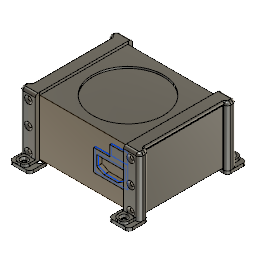
PSU (Autodesk Fusion 360 design; units mm, degrees)
Autodesk Fusion 360 part; units mm, degrees
sketch "Sketch1" plane through (0, 0, 0) normal (0, 0, 1) x (1, 0, 0)
  line L0 (50, 50) -> (-50, 50) construction
  line L1 (-50, 50) -> (-50, -50) construction
  line L2 (-50, -50) -> (50, -50) construction
  line L3 (50, -50) -> (50, 50) construction
  line L4 (50, 50) -> (-50, -50) construction
  line L5 (-50, 50) -> (50, -50) construction
  circle A0 centre (-50, -50) radius 2.25
  circle A1 centre (-50, -50) radius 3.75
  circle A2 centre (50, -50) radius 3.75
  circle A3 centre (50, -50) radius 2.25
  circle A4 centre (50, 50) radius 3.75
  circle A5 centre (50, 50) radius 2.25
  circle A6 centre (-50, 50) radius 3.75
  circle A7 centre (-50, 50) radius 2.25
  line L6 (63, 50.5) -> (-63, 50.5) construction
  line L7 (-63, 50.5) -> (-63, -50.5)
  line L8 (-63, -50.5) -> (63, -50.5)
  line L9 (63, -50.5) -> (63, 50.5) construction
  line L10 (63, 50.5) -> (-63, -50.5) construction
  line L11 (-63, 50.5) -> (63, -50.5) construction
  line L12 (-50, -50) -> (-63, -50) construction
  line L13 (-56.5, -50) -> (-56.5, -61) construction
  circle A8 centre (-56.5, -61) radius 2.25
  line L14 (-56.5, -61) -> (-50, -50) construction
  line L15 (-48.4461, -44.5539) -> (-64, -44.5539)
  line L16 (-68, -48.5539) -> (-68, -62.9425)
  line L17 (-64, -66.9425) -> (-48.4461, -66.9425)
  line L18 (-44.4461, -62.9425) -> (-44.4461, -48.5539)
  arc A9 (-68, -62.9425) -> (-64, -66.9425) centre (-64, -62.9425) ccw
  arc A10 (-44.4461, -48.5539) -> (-48.4461, -44.5539) centre (-48.4461, -48.5539) ccw
  arc A11 (-48.4461, -66.9425) -> (-44.4461, -62.9425) centre (-48.4461, -62.9425) ccw
  arc A12 (-64, -44.5539) -> (-68, -48.5539) centre (-64, -48.5539) ccw
  line L19 (-56.4568, -56.7278) -> (-60.1782, -58.8265)
  line L20 (-60.1782, -58.8265) -> (-60.2214, -63.0987)
  line L21 (-60.2214, -63.0987) -> (-56.5432, -65.2722)
  line L22 (-56.5432, -65.2722) -> (-52.8218, -63.1735)
  line L23 (-52.8218, -63.1735) -> (-52.7786, -58.9013)
  line L24 (-52.7786, -58.9013) -> (-56.4568, -56.7278)
  circle A13 centre (-50, -50) radius 4.5
  point P0 (-53.25, -55.5)
  point P1 (-53.25, -55.5)
  point P2 (-56.5, -61)
  dimension "d1" = 100
  dimension "d2" = 100
  dimension "d3" = 4.5
  dimension "d4" = 7.5
  dimension "d6" = 360
  dimension "d7" = 126
  dimension "d8" = 101
  dimension "d9" = 11
  dimension "d10" = 4.5
  dimension "d11" = 4
  dimension "d12" = 3.7
  dimension "d23" = 5
  dimension "d24" = 9
  constraint perpendicular L0 L1
  constraint parallel L0 L2
  constraint parallel L1 L3
  constraint horizontal L0
  constraint coincident L4 origin
  constraint coincident L5 origin
  constraint coincident L1.end L2.start
  constraint concentric A0 A1
  constraint perpendicular L6 L7
  constraint parallel L6 L8
  constraint parallel L7 L9
  constraint horizontal L6
  constraint coincident L10 origin
  constraint coincident L11 origin
  constraint coincident L7 L12.end
  constraint perpendicular L7 L12
  constraint midpoint L12 L13.start
  constraint perpendicular L8 L13
  constraint coincident P2 L13.end
  constraint midpoint L14 P1
  constraint perpendicular L15 L16
  constraint parallel L15 L17
  constraint parallel L16 L18
  constraint horizontal L15
  constraint coincident P1 P0
  constraint tangent L16 A9
  constraint tangent L17 A9
  constraint tangent L15 A10
  constraint tangent L18 A10
  constraint equal A9 A10
  constraint tangent L18 A11
  constraint tangent L17 A11
  constraint equal A9 A11
  constraint tangent L15 A12
  constraint tangent L16 A12
  constraint equal A9 A12
  measures "d1" distance of L1.end L2.end
  measures "d2" distance of L0.end L1.end
  measures "d3" diameter of A0
  measures "d4" diameter of A1
  measures "d7" distance of L7.end L8.end
  measures "d8" distance of L6.end L7.end
  measures "d9" distance of L13.start P2
  measures "d10" diameter of A8
  measures "d11" radius of A9
  measures "d12" distance of P2 L24
  measures "d23" distance of L7 L16
  measures "d24" diameter of A13
extrude "Extrude1" add sketch "Sketch1" against normal blind 1 contours A1 L8 A13 | A1 L8 A13 | L7 L8 L15 L16 L17 L18 A9 A11 A12 A13 | L7 L8 L15 L18 A10 A13 makes body 1
extrude "Extrude2" add sketch "Sketch1" along normal blind 1 contours A0 A1 L8 | A0 A1 L8 | A1 L8 A13 | A1 L8 A13 | L7 L8 L15 L16 L17 L18 A9 A11 A12 A13 | L7 L8 L15 L18 A10 A13 bodies 1
extrude "Extrude3" add sketch "Sketch1" along normal blind 1.5 from surface at 1 contours L7 L8 L15 L16 L17 L18 A9 A11 A12 A13 | L7 L8 L15 L18 A10 A13 | L19 L20 L21 L22 L23 L24 bodies 1
mirror "Mirror1" about plane through (0, 0, 0) normal (0, 1, 0) of bodies 1 makes body 2
sketch "Sketch2" plane through (0, 0, 2.5) normal (0, 0, 1) x (-1, 0, 0)
  circle A0 centre (56.5, 61) radius 2.25
  circle A1 centre (50, 50) radius 4.5
  arc A2 (64, 44.5539) -> (68, 48.5539) centre (64, 48.5539) ccw
  line L0 (68, 48.5539) -> (68, 62.9425)
  arc A3 (68, 62.9425) -> (64, 66.9425) centre (64, 62.9425) ccw
  line L1 (64, 66.9425) -> (48.4461, 66.9425)
  arc A4 (48.4461, 66.9425) -> (44.4461, 62.9425) centre (48.4461, 62.9425) ccw
  line L2 (44.4461, 62.9425) -> (44.4461, 48.5539)
  arc A5 (44.4461, 48.5539) -> (48.4461, 44.5539) centre (48.4461, 48.5539) ccw
  line L3 (48.4461, 44.5539) -> (64, 44.5539)
  line L4 (63, -50.5) -> (63, 50.5)
  line L5 (63, 50.5) -> (-63, 50.5)
  line L6 (54.9957, 66.9425) -> (57.9957, 66.9425)
  line L7 (62.9957, 61.9425) -> (62.9957, 56.0653)
  line L8 (49.9957, 55.0496) -> (49.9957, 61.9425)
  line L9 (49.9957, 66.9425) -> (62.9957, 55.0653) construction
  line L10 (62.9957, 66.9425) -> (49.9957, 55.0496) construction
  line L11 (64, 66.9425) -> (48.4461, 66.9425)
  line L12 (63.9957, 55.0653) -> (63.9997, 55.0653)
  line L13 (49.9957, 55.0496) -> (49.9957, 50.5)
  arc A6 (62.9957, 56.0653) -> (63.9957, 55.0653) centre (63.9957, 56.0653) ccw
  line L14 (67.9997, 51.0657) -> (68, 48.5539)
  arc A7 (67.9997, 51.0657) -> (63.9997, 55.0653) centre (63.9997, 51.0653) ccw
  arc A8 (62.9957, 61.9425) -> (57.9957, 66.9425) centre (57.9957, 61.9425) ccw
  arc A9 (54.9957, 66.9425) -> (49.9957, 61.9425) centre (54.9957, 61.9425) ccw
  line L15 (63.9997, 55.0653) -> (49.9957, 55.0496)
  point P0 (56.5, 61)
  dimension "d25" = 13
  dimension "d26" = 1
  dimension "d27" = 4
  dimension "d28" = 5
  constraint perpendicular L6 L7
  constraint parallel L7 L8
  constraint horizontal L6
  constraint coincident L9 P0
  constraint coincident L10 P0
  constraint coincident P0 A0.centre
  constraint collinear L6 L11
  constraint perpendicular L0 L12
  constraint coincident L5 L13.end
  constraint perpendicular L5 L13
  constraint coincident L9.end L12
  constraint coincident L9.end L7
  constraint tangent L12 A6
  constraint tangent L7 A6
  constraint coincident A2.end L0.start
  constraint tangent L12 A7
  constraint tangent L14 A7
  constraint coincident L10.start L7
  constraint coincident L10.start L6
  constraint tangent L7 A8
  constraint tangent L6 A8
  constraint coincident L9.start L8
  constraint coincident L9.start L6
  constraint tangent L8 A9
  constraint tangent L6 A9
  constraint equal A8 A9
  measures "d25" distance of L9.end L8.start
  measures "d26" radius of A6
  measures "d27" radius of A7
  measures "d28" radius of A8
extrude "Extrude4" add sketch "Sketch2" along normal blind 3 separate body contours A1 L5 L13 | A1 A2 L0 L3 L4 L5 L12 L13 L14 A7 L15 | L1 L6 L7 L8 L11 A6 A8 A9 L15 picked at (52.9399, 50.7152) makes body 3
extrude "Extrude5" add sketch "Sketch2" along normal blind 67 contours A1 L5 L13 | A1 A2 L0 L3 L4 L5 L12 L13 L14 A7 L15 picked at (52.9399, 50.7152) bodies 3
mirror "Mirror2" about plane through (0, 0, 0) normal (0, 1, 0) of bodies 3 makes body 4
sketch "Sketch3" plane through (0.0616, -54.9935, 0) normal (0.001121, -0.999999, 0) x (0.999999, 0.001121, 0)
  line L0 (-64.0574, 5.5) -> (-50.0574, 5.5)
  line L1 (-50.0574, 5.5) -> (-50.0574, 69.5)
  line L2 (-50.0574, 69.5) -> (-64.0614, 69.5)
  line L3 (-64.0614, 69.5) -> (-64.0614, 2.5)
  line L4 (-50.0574, 69.5) -> (-64.0614, 69.5)
  line L5 (-64.0614, 69.5) -> (-64.0614, 66.5)
  line L6 (-64.0614, 66.5) -> (-50.0574, 66.5)
  line L7 (-50.0574, 66.5) -> (-50.0574, 69.5)
  line L8 (-58.0614, 66.5) -> (-58.0614, 5.5) construction
  circle A0 centre (-58.0614, 60.5) radius 2.25
  circle A1 centre (-58.0614, 34.7) radius 2.25
  circle A2 centre (-58.0614, 9) radius 2.25
  line L9 (-64.0574, 2.5) -> (-64.0574, 5.5)
  line L10 (-64.0614, 2.5) -> (-64.0574, 2.5)
  dimension "d34" = 3
  dimension "d37" = 6
  dimension "d38" = 4.5
  dimension "d39" = 4.5
  dimension "d40" = 4.5
  dimension "d41" = 6
  dimension "d42" = 25.8
  dimension "d43" = 51.5
  constraint horizontal L4
  constraint vertical L5
  constraint horizontal L6
  constraint vertical L7
  constraint coincident L1.end L2.start
  constraint coincident L6 L8.start
  constraint coincident L0 L8.end
  constraint perpendicular L0 L8
  constraint coincident L8 A0.centre
  constraint coincident L8 A1.centre
  constraint coincident L8 A2.centre
  measures "d34" distance of L1.end L6.end
  measures "d37" distance of L3 L8
  measures "d38" diameter of A0
  measures "d39" diameter of A1
  measures "d40" diameter of A2
  measures "d41" distance of L6 A0.centre
  measures "d42" distance of A0.centre A1.centre
  measures "d43" distance of A0.centre A2.centre
extrude "Extrude6" add sketch "Sketch3" against normal blind 110 contours L1 L2 L3 L4 L5 L6 L7 bodies 3 4
extrude "Extrude7" cut sketch "Sketch3" against normal blind 10 contours A0 | A1 | A2 bodies 3
fillet "Fillet1" radius 3 4 edges at (-66.8325, -45.7295, 69.5) (-67.9999, -49.8098, 69.5) (-66.828, -53.8939, 69.5) (-56.9977, -55.0575, 69.5) on bodies 3
fillet "Fillet1" radius 2 1 edges at (-64.0614, 0.0008, 69.5) on bodies 3
fillet "Fillet1" radius 3 4 edges at (-66.8675, 45.7651, 69.5) (-67.9999, 49.8098, 69.5) (-66.828, 53.8939, 69.5) (-56.9977, 55.0575, 69.5) on bodies 3
chamfer "Chamfer1" distance 2 angle 45 5 edges at (-54.4023, -61.8136, 5.5) (-60.0975, -55.0609, 9.8136) (-60.0975, -55.0609, 35.5136) (-60.0975, -55.0609, 61.3136) (-54.4023, 61.8136, 5.5) on bodies 3 4
mirror "Mirror3" about plane through (0, 0, 0) normal (1, 0, 0) of bodies 3 1 2 makes body 5 at (54.0272, 15.0364, 66.5) makes body 6 at (64.7863, 57.0763, 2.5) makes body 7 at (64.7863, -57.0763, 2.5)
sketch "Sketch4" plane through (0, 0, 66.5) normal (0, 0, -1) x (1, 0, 0)
  arc A0 (-64, -44.5539) -> (-64.1114, -44.5555) centre (-64, -48.5539) ccw
  line L0 (-64, -44.5539) -> (-63, -44.5539)
  line L1 (-63, -44.5539) -> (-63, -50.5)
  line L2 (-63, -50.5) -> (-50.114, -50.5)
  line L3 (-50.114, -50.5) -> (-50.0008, 50.5)
  line L4 (-50.0008, 50.5) -> (-63, 50.5)
  line L5 (-63, 50.5) -> (-63, 44.5539)
  line L6 (-63, 44.5539) -> (-64, 44.5539)
  arc A1 (-64.0115, 44.5539) -> (-64, 44.5539) centre (-64, 48.5539) ccw
  line L7 (-64.0115, 44.5539) -> (-64.1114, -44.5555)
  line L8 (62.5, 50) -> (-62.5, 50)
  line L9 (-62.5, 50) -> (-62.5, -50)
  line L10 (-62.5, -50) -> (62.5, -50)
  line L11 (62.5, -50) -> (62.5, 50)
  line L12 (62.5, 50) -> (-62.5, -50) construction
  line L13 (-62.5, 50) -> (62.5, -50) construction
  circle A2 centre (0, 0) radius 40
  dimension "d51" = 100
  dimension "d52" = 125
  dimension "d55" = 80
  constraint perpendicular L8 L9
  constraint parallel L8 L10
  constraint parallel L9 L11
  constraint horizontal L8
  constraint coincident L12 A2.centre
  constraint coincident L13 A2.centre
  constraint coincident A2.centre origin
  measures "d51" distance of L8.end L9.end
  measures "d52" distance of L9.end L10.end
  measures "d55" diameter of A2
extrude "Extrude8" add sketch "Sketch4" along normal blind 63 separate body contours L3 L8 L9 L10 | L3 L8 L10 L11 | A2 makes body 8
extrude "Extrude9" cut sketch "Sketch4" along normal blind 2 contours A2 bodies 8
sketch "Sketch5" plane through (0, -50, 0) normal (0, -1, 0) x (1, 0, 0)
  line L0 (62.5, 66.5) -> (-62.5, 66.5)
  line L1 (-62.5, 66.5) -> (-62.5, 3.5)
  line L2 (-62.5, 3.5) -> (62.5, 3.5)
  line L3 (62.5, 3.5) -> (62.5, 66.5)
  line L4 (49.8097, 23.1578) -> (12.951, 23.1578)
  line L5 (12.951, 23.1578) -> (12.951, 47.6426)
  line L6 (12.951, 47.6426) -> (49.8097, 47.6426)
  line L7 (49.8097, 47.6426) -> (49.8097, 23.1578)
  line L8 (31.3803, 47.6426) -> (49.8097, 47.6426)
  line L9 (49.8097, 47.6426) -> (49.8097, 59.7533)
  line L10 (49.8097, 59.7533) -> (31.3803, 59.7533)
  line L11 (31.3803, 59.7533) -> (31.3803, 47.6426)
  line L12 (16.5299, 42.2654) -> (16.5299, 30.7332)
  line L13 (16.5299, 30.7332) -> (24.6911, 26.6526)
  line L14 (24.6911, 26.6526) -> (40.595, 26.6526)
  line L15 (40.595, 26.6526) -> (46.8685, 30.7332)
  line L16 (46.8685, 30.7332) -> (46.8685, 42.2654)
  line L17 (46.8685, 42.2654) -> (16.5299, 42.2654)
  constraint horizontal L4
  constraint vertical L5
  constraint horizontal L6
  constraint vertical L7
  constraint horizontal L8
  constraint vertical L9
  constraint horizontal L10
  constraint vertical L11
  constraint midpoint L6 L8.start
  constraint collinear L7 L9
  constraint perpendicular L6 L12
  constraint parallel L6 L14
  constraint parallel L12 L16
  constraint perpendicular L12 L17
extrude "Extrude10" add sketch "Sketch5" along normal blind 2 contours L4 L5 L6 L7 L8 | L6 L8 L9 L10 L11 | L12 L13 L14 L15 L16 L17 bodies 8
extrude "Extrude11" cut sketch "Sketch5" along normal mid plane 8 contours L12 L13 L14 L15 L16 L17 bodies 8
named bodies: "VESA1", "VESA2", "PSU1", "PSU2", "VESA4", "PSU", "VESA3"
